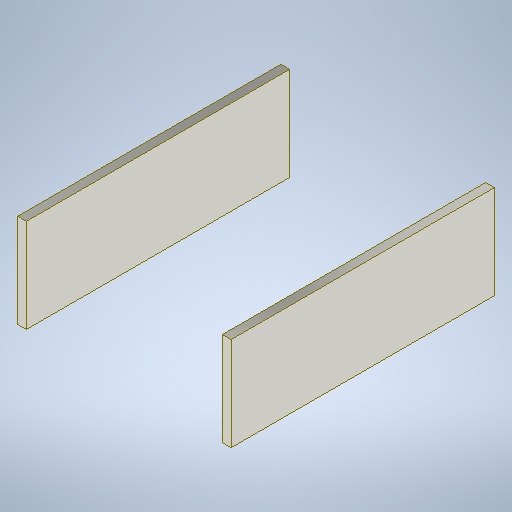
# Autodesk Inventor part: Eslabón2_Largo
Saved by Autodesk Inventor 2025.1 (Build 291241000, 241)
## iProperties
Created: 2024-12-02
Part Number: Eslabón2_Largo
Material: Stainless Steel
Document SubType Name: Modeling
Designer: Cristhian Vigo
Density: 7.60422 g/cm^3
Appearance: Silver
Author: Cristhian Vigo
Autodesk Inventor part; units mm, degrees
ref_plane "YZ Plane" through (0, 0, 0) normal (1, 0, 0) x (0, 1, 0)
ref_plane "XZ Plane" through (0, 0, 0) normal (0, 1, 0) x (-1, 0, 0)
ref_plane "XY Plane" through (0, 0, 0) normal (0, 0, 1) x (1, 0, 0)
sketch "Sketch1" plane through (0, 0, 0) normal (0, 0, 1) x (1, 0, 0)
  line L0 (-36.5, 16) -> (36.5, 16) construction
  line L1 (-36.5, 16) -> (-33.5, 16)
  line L2 (-33.5, 16) -> (-33.5, -16)
  line L3 (-33.5, -16) -> (-36.5, -16)
  line L4 (-36.5, -16) -> (-36.5, 16)
  line L5 (0, 16) -> (0, -16) construction
  line L6 (36.5, 16) -> (33.5, 16)
  line L7 (33.5, 16) -> (33.5, -16)
  line L8 (33.5, -16) -> (36.5, -16)
  line L9 (36.5, -16) -> (36.5, 16)
  point P0 (0, 0)
  dimension "d0" = 73
  dimension "d1" = 3
  dimension "d2" = 32
  dimension "d3" = 16
  constraints: 20 end point, 3 symmetric about line, 2 horizontal, 2 parallel, 1 midpoint, 1 perpendicular, 1 vertical, 1 vertical alignment
  measures "d0" distance of L0.start L0.end
  measures "d1" distance of L2.end L3.end
  measures "d2" distance of L1.end L2.end
  measures "d3" distance of L5.start point (0, 0)
extrude "Extrusion1" add sketch "Sketch1" along normal blind 90
equation "\"d0\" = Esla_Bas_Largo"
equation "\"d1\" = Esla_Bas_Espesor"
equation "\"d2\" = Esla_Bas_Ancho"
equation "\"Esla_Bas_Largo\" = 73"
equation "\"Esla_Bas_Espesor\" = 3"
equation "\"Esla_Bas_Ancho\" = 32"
body "Solid1"
